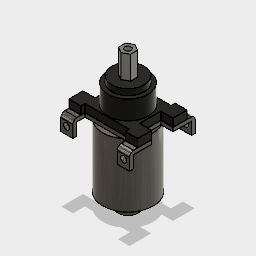
Motor (Autodesk Fusion 360 design; units mm, degrees)
Autodesk Fusion 360 part; units mm, degrees
sketch "Sketch1" plane through (0, 0, 0) normal (0, 1, 0) x (1, 0, 0)
  circle A0 centre (0, 0) radius 5
extrude "Extrude1" add sketch "Sketch1" along normal blind 6.8 makes body 1
sketch "Sketch2" plane through (0, 6.8, 0) normal (0, 1, 0) x (-1, 0, 0)
  circle A0 centre (0, 0) radius 5
  circle A1 centre (0, 0) radius 12.5
  dimension "d3" = 25
  measures "d3" diameter of A1
extrude "Extrude2" add sketch "Sketch2" along normal blind 31.4 contours A0 | A1 bodies 1
sketch "Sketch3" plane through (0, 38.2, 0) normal (0, 1, 0) x (-1, 0, 0)
  circle A0 centre (0, 0) radius 12.5
  line L0 (-11, -10.25) -> (11, -10.25)
  line L1 (11, -10.25) -> (11, 10.25)
  line L2 (11, 10.25) -> (-11, 10.25)
  line L3 (-11, 10.25) -> (-11, -10.25)
  line L4 (-11, -10.25) -> (11, 10.25) construction
  line L5 (11, -10.25) -> (-11, 10.25) construction
  line L6 (-11, -10.25) -> (-11, -16.25)
  line L7 (-11, -16.25) -> (-17, -16.25)
  line L8 (-17, -16.25) -> (-17, -5.25)
  line L9 (-17, -5.25) -> (-11, -5.25)
  line L10 (-11, 10.25) -> (-11, 16.25)
  line L11 (-11, 16.25) -> (-17, 16.25)
  line L12 (-17, 16.25) -> (-17, 5.25)
  line L13 (-17, 5.25) -> (-11, 5.25)
  line L14 (11, 10.25) -> (11, 16.25)
  line L15 (11, 16.25) -> (17, 16.25)
  line L16 (17, 16.25) -> (17, 5.25)
  line L17 (17, 5.25) -> (11, 5.25)
  line L18 (11, -10.25) -> (11, -16.25)
  line L19 (11, -16.25) -> (17, -16.25)
  line L20 (17, -16.25) -> (17, -5.25)
  line L21 (17, -5.25) -> (11, -5.25)
  dimension "d39" = 22
  dimension "d44" = 20.5
  dimension "d45" = 6
  dimension "d46" = 6
  dimension "d47" = 11
  dimension "d48" = 6
  dimension "d49" = 6
  dimension "d50" = 11
  dimension "d51" = 6
  dimension "d52" = 6
  dimension "d53" = 11
  dimension "d54" = 6
  dimension "d55" = 6
  dimension "d56" = 11
  measures "d39" distance of L1 L3
  measures "d44" distance of L0.start L2.end
  measures "d45" distance of L0.start L6.end
  measures "d46" distance of L6.end L7.end
  measures "d47" distance of L7.end L8.end
  measures "d48" distance of L2.end L10.end
  measures "d49" distance of L10.end L11.end
  measures "d50" distance of L11.end L12.end
  measures "d51" distance of L1.end L14.end
  measures "d52" distance of L14.end L15.end
  measures "d53" distance of L15.end L16.end
  measures "d54" distance of L0.end L18.end
  measures "d55" distance of L18.end L19.end
  measures "d56" distance of L19.end L20.end
extrude "Extrude3" add sketch "Sketch3" along normal blind 1.9 separate body contours A0 L1 L17 | A0 L1 L14 L15 L16 L17 | A0 L1 L18 L19 L20 L21 | A0 L1 L21 | A0 L0 L1 L2 L3 | A0 L1 L2 | A0 L0 L1 | A0 L2 L3 | A0 L0 L3 | A0 L3 L13 | A0 L3 L10 L11 L12 L13 | A0 L3 L6 L7 L8 L9 | A0 L3 L9 makes body 2
sketch "Sketch4" plane through (0, 38.2, 0) normal (0, -1, 0) x (1, 0, 0)
  line L0 (-17, 16.25) -> (-11, 16.25)
  line L1 (-11, 16.25) -> (-11, 14.35)
  line L2 (-11, 14.35) -> (-17, 14.35)
  line L3 (-17, 14.35) -> (-17, 16.25)
  line L4 (11, 16.25) -> (17, 16.25)
  line L5 (17, 16.25) -> (17, 14.35)
  line L6 (17, 14.35) -> (11, 14.35)
  line L7 (11, 14.35) -> (11, 16.25)
  line L8 (17, -16.25) -> (11, -16.25)
  line L9 (11, -16.25) -> (11, -14.35)
  line L10 (11, -14.35) -> (17, -14.35)
  line L11 (17, -14.35) -> (17, -16.25)
  line L12 (-17, -16.25) -> (-11, -16.25)
  line L13 (-11, -16.25) -> (-11, -14.35)
  line L14 (-11, -14.35) -> (-17, -14.35)
  line L15 (-17, -14.35) -> (-17, -16.25)
  point P0 (-17, 16.25)
  point P1 (11, 16.25)
  point P2 (17, -16.25)
  point P3 (-17, -16.25)
  dimension "d57" = 1.9
  dimension "d58" = 1.9
  dimension "d59" = 1.9
  dimension "d60" = 1.9
  measures "d57" distance of P0 L2.end
  measures "d58" distance of P1 L6.end
  measures "d59" distance of P2 L10.end
  measures "d60" distance of P3 L14.end
extrude "Extrude4" add sketch "Sketch4" along normal blind 6.1 bodies 1 2
fillet "Fillet1" radius 2 4 edges at (-14, 40.1, 16.25) (14, 40.1, 16.25) (-14, 40.1, -16.25) (14, 40.1, -16.25) on bodies 2
sketch "Sketch5" plane through (0, 0, -16.25) normal (0, 0, -1) x (-1, 0, 0)
  line L0 (12.5, 6.8) -> (-12.5, 6.8)
  line L1 (0, 6.8) -> (0, 35.75)
  line L2 (0, 35.75) -> (14.1, 35.75)
  line L3 (0, 35.75) -> (-14.1, 35.75)
  circle A0 centre (-14.1, 35.75) radius 1.5
  circle A1 centre (14.1, 35.75) radius 1.5
  dimension "d62" = 28.95
  dimension "d63" = 14.1
  dimension "d64" = 14.1
  dimension "d65" = 3
  dimension "d66" = 3
  measures "d62" distance of L1.start L1.end
  measures "d63" distance of L1.end L2.end
  measures "d64" distance of L1.end L3.end
  measures "d65" diameter of A0
  measures "d66" diameter of A1
extrude "Extrude5" cut sketch "Sketch5" against normal blind 51 bodies 1 2
sketch "Sketch6" plane through (0, 40.1, 0) normal (0, 1, 0) x (-1, 0, 0)
  line L0 (17, -5.25) -> (11, -5.25)
  line L1 (17, -5.25) -> (11, -5.25)
  line L2 (11, -5.25) -> (11, 5.25)
  line L3 (11, 5.25) -> (17, 5.25)
  line L4 (11, -10.25) -> (-11, -10.25)
  line L5 (-11, -5.25) -> (-11, 5.25)
  line L6 (-11, -5.25) -> (-17, -5.25)
  line L7 (-11, -5.25) -> (-11, 5.25)
  line L8 (-11, 5.25) -> (-17, 5.25)
  line L9 (-17, 5.25) -> (-17, 12.25)
  line L10 (-11, 10.25) -> (-11, 14.25)
  line L11 (-17, 12.25) -> (-11, 12.25)
  line L12 (-11, 12.25) -> (-11, 10.25)
  line L13 (-11, 10.25) -> (11, 10.25)
  line L14 (17, 5.25) -> (17, 12.25)
  line L15 (11, 14.25) -> (11, 10.25)
  line L16 (17, 12.25) -> (11, 12.25)
  line L17 (11, 12.25) -> (11, 10.25)
  line L18 (17, -5.25) -> (17, -12.25)
  line L19 (11, -10.25) -> (11, -14.35)
  line L20 (17, -12.25) -> (11, -12.3)
  line L21 (11, -12.3) -> (11, -10.25)
  line L22 (-17, -5.25) -> (-17, -12.25)
  line L23 (-11, -14.25) -> (-11, -10.25)
  line L24 (-17, -12.25) -> (-11, -12.25)
  line L25 (-11, -12.25) -> (-11, -10.25)
  point P0 (17, -5.25)
  point P1 (11, -5.25)
  point P2 (11, -5.25)
  point P3 (11, 5.25)
  point P4 (17, 5.25)
  point P5 (11, -10.25)
  point P6 (-11, -10.25)
  point P7 (-11, -5.25)
  point P8 (-17, -5.25)
  point P9 (-17, 5.25)
  point P10 (11, 10.25)
  dimension "d67" = 7
  dimension "d68" = 7
  dimension "d69" = 7
  dimension "d70" = 7
  measures "d67" distance of P9 L9.end
  measures "d68" distance of P4 L14.end
  measures "d69" distance of P0 L18.end
  measures "d70" distance of P8 L22.end
extrude "Extrude6" add sketch "Sketch6" along normal blind 4 separate body makes body 3
sketch "Sketch7" plane through (0, 44.1, 0) normal (0, 1, 0) x (-1, 0, 0)
  circle A0 centre (0, 0) radius 10
  line L0 (-11, -5.25) -> (-17, -5.25)
  line L1 (-17, -5.25) -> (-17, -12.25)
  line L2 (-17, -12.25) -> (-11, -12.25)
  line L3 (-11, -12.25) -> (-11, -10.25)
  line L4 (11, -10.25) -> (11, -12.3)
  line L5 (11, -12.3) -> (17, -12.25)
  line L6 (17, -12.25) -> (17, -5.25)
  line L7 (17, -5.25) -> (11, -5.25)
  line L8 (11, 5.25) -> (17, 5.25)
  line L9 (17, 5.25) -> (17, 12.25)
  line L10 (17, 12.25) -> (11, 12.25)
  line L11 (11, 12.25) -> (11, 10.25)
  line L12 (-11, 10.25) -> (-11, 12.25)
  line L13 (-11, 12.25) -> (-17, 12.25)
  line L14 (-17, 12.25) -> (-17, 5.25)
  line L15 (-17, 5.25) -> (-11, 5.25)
  line L16 (-11, -10.25) -> (11, -10.25)
  line L17 (11, -5.25) -> (11, 5.25)
  line L18 (11, 10.25) -> (-11, 10.25)
  line L19 (-11, 5.25) -> (-11, -5.25)
  dimension "d25" = 20
  measures "d25" diameter of A0
extrude "Extrude7" add sketch "Sketch7" along normal blind 9.4 contours A0 bodies 3
sketch "Sketch8" plane through (0, 53.5, 0) normal (0, 1, 0) x (-1, 0, 0)
  circle A0 centre (0, 0) radius 10
  circle A1 centre (0, 0) radius 8
extrude "Extrude8" add sketch "Sketch8" along normal blind 3 contours A1 bodies 1 makes body 4
sketch "Sketch9" plane through (0, 56.5, 0) normal (0, 1, 0) x (-1, 0, 0)
  circle A0 centre (0, 0) radius 8
  line L0 (0, -3.5) -> (3.0311, -1.75)
  line L1 (3.0311, -1.75) -> (3.0311, 1.75)
  line L2 (3.0311, 1.75) -> (0, 3.5)
  line L3 (0, 3.5) -> (-3.0311, 1.75)
  line L4 (-3.0311, 1.75) -> (-3.0311, -1.75)
  line L5 (-3.0311, -1.75) -> (0, -3.5)
extrude "Extrude9" add sketch "Sketch9" along normal blind 11.5 separate body contours L0 L1 L2 L3 L4 L5 makes body 5
sketch "Sketch10" plane through (0, 68, 0) normal (0, 1, 0) x (-1, 0, 0)
  line L0 (-3.0311, -1.75) -> (0, -3.5)
  line L1 (0, -3.5) -> (3.0311, -1.75)
  line L2 (3.0311, -1.75) -> (3.0311, 1.75)
  line L3 (3.0311, 1.75) -> (0, 3.5)
  line L4 (0, 3.5) -> (-3.0311, 1.75)
  line L5 (-3.0311, 1.75) -> (-3.0311, -1.75)
  circle A0 centre (0, 0) radius 1.5
  dimension "d32" = 3
  measures "d32" diameter of A0
extrude "Extrude10" cut sketch "Sketch10" against normal blind 5 contours A0 bodies 4 5 1
